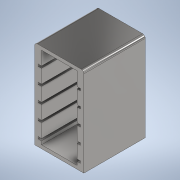
# Autodesk Inventor part: RackV2
Saved by Autodesk Inventor 2021 (Build 250183000, 183)
## iProperties
Created: 2023-04-06
Part Number: RackV2
Material: Steel
Document SubType Name: Modeling
Designer: EF0481
Density: 7.85 g/cm^3
Appearance: Steel - Polished
Author: EF0481
Autodesk Inventor part; units mm, degrees
ref_plane "YZ Plane" through (0, 0, 0) normal (1, 0, 0) x (0, 1, 0)
ref_plane "XZ Plane" through (0, 0, 0) normal (0, 1, 0) x (-1, 0, 0)
ref_plane "XY Plane" through (0, 0, 0) normal (0, 0, 1) x (1, 0, 0)
sketch "Sketch1" plane through (0, 0, 0) normal (0, 0, 1) x (1, 0, 0)
  line L0 (0, 0) -> (72, 0)
  line L1 (72, 0) -> (72, 130)
  line L2 (72, 130) -> (0, 130)
  line L3 (0, 130) -> (0, 0)
  dimension "d0" = 72
  dimension "d1" = 130
  constraints: 8 end point, 2 parallel, 1 horizontal, 1 perpendicular
  measures "d0" distance of L2.end L1.end
  measures "d1" distance of L1.end L0.end
extrude "Extrusion1" add sketch "Sketch1" along normal blind 90
sketch "Sketch2" plane through (0, 0, 90) normal (0, 0, 1) x (1, 0, 0)
  line L0 (10, 125) -> (10, 105)
  line L1 (10, 105) -> (5, 105)
  line L2 (5, 105) -> (5, 102)
  line L3 (5, 102) -> (10, 102)
  line L4 (10, 102) -> (10, 82)
  line L5 (10, 82) -> (5, 82)
  line L6 (5, 82) -> (5, 79)
  line L7 (5, 79) -> (10, 79)
  line L8 (10, 79) -> (10, 59)
  line L9 (10, 59) -> (5, 59)
  line L10 (5, 59) -> (5, 56)
  line L11 (5, 56) -> (10, 56)
  line L12 (10, 56) -> (10, 36)
  line L13 (10, 36) -> (5, 36)
  line L14 (5, 36) -> (5, 33)
  line L15 (5, 33) -> (10, 33)
  line L16 (10, 33) -> (10, 13)
  line L17 (10, 13) -> (5, 13)
  line L18 (5, 13) -> (5, 10)
  line L19 (5, 10) -> (10, 10)
  line L20 (10, 79.6722) -> (10, 76.6722)
  line L21 (10, 125) -> (62, 125) projected
  line L22 (62, 5) -> (10, 5) projected
  line L23 (62, 105) -> (67, 105)
  line L24 (67, 105) -> (67, 102)
  line L25 (67, 102) -> (62, 102)
  line L26 (62, 82) -> (67, 82)
  line L27 (67, 82) -> (67, 79)
  line L28 (67, 79) -> (62, 79)
  line L29 (62, 59) -> (67, 59)
  line L30 (67, 59) -> (67, 56)
  line L31 (67, 56) -> (62, 56)
  line L32 (62, 36) -> (67, 36)
  line L33 (67, 36) -> (67, 33)
  line L34 (67, 33) -> (62, 33)
  line L35 (62, 13) -> (67, 13)
  line L36 (67, 13) -> (67, 10)
  line L37 (67, 10) -> (62, 10)
  line L38 (10, 125) -> (62, 125)
  line L39 (62, 125) -> (62, 105)
  line L40 (62, 102) -> (62, 82)
  line L41 (62, 79) -> (62, 59)
  line L42 (62, 56) -> (62, 36)
  line L43 (62, 33) -> (62, 13)
  line L44 (62, 10) -> (62, 5)
  line L45 (10, 10) -> (10, 5)
  point P0 (0, 0)
  dimension "d7" = 20
  dimension "d8" = 5
  dimension "d9" = 3
  dimension "d10" = 20
  dimension "d11" = 5
  dimension "d12" = 3
  dimension "d13" = 20
  dimension "d14" = 3
  dimension "d15" = 20
  dimension "d16" = 5
  dimension "d17" = 3
  dimension "d18" = 20
  dimension "d19" = 3
  dimension "d20" = 3
  constraints: 88 end point, 8 perpendicular, 6 point on line, 4 collinear, 3 vertical, 1 horizontal
  measures "d7" distance of L0.start L0.end
  measures "d8" distance of L0.end L1.end
  measures "d9" distance of L1.end L2.end
  measures "d10" distance of L3.end L4.end
  measures "d11" distance of L4.end L5.end
  measures "d12" distance of L5.end L6.end
  measures "d13" distance of L7.end L8.end
  measures "d14" distance of L9.end L10.end
  measures "d15" distance of L11.end L12.end
  measures "d16" distance of L12.end L13.end
  measures "d17" distance of L13.end L14.end
  measures "d18" distance of L15.end L16.end
  measures "d19" distance of L17.end L18.end
  measures "d20" distance of L20.start L20.end
extrude "Extrusion2" cut sketch "Sketch2" against normal blind 90
fillet "Fillet1" radius 4 2 edges at (72, 130, 45) (0, 130, 45)
sketch "Sketch3" plane through (0, 0, 0) normal (0, 0, -1) x (-1, 0, 0)
  circle A0 centre (-67, 125) radius 1.5
  line L0 (-72, 126) -> (-72, 0)
  line L1 (-4, 130) -> (-68, 130)
  line L2 (0, 0) -> (0, 126)
  arc A1 (0, 126) -> (-4, 130) centre (-4, 126) ccw
  line L3 (-4, 130) -> (-68, 130)
  arc A2 (-68, 130) -> (-72, 126) centre (-68, 126) ccw
  line L4 (-72, 126) -> (-72, 0)
  line L5 (-72, 0) -> (0, 0)
  line L6 (0, 0) -> (0, 126)
  line L7 (-68, 130) -> (-4, 130)
  line L8 (0, 0) -> (-72, 0)
  circle A3 centre (-5, 125) radius 1.5
  circle A4 centre (-67, 5) radius 1.5
  circle A5 centre (-5, 5) radius 1.5
  dimension "d24" = 3
  dimension "d25" = 5
  dimension "d26" = 5
  dimension "d27" = 3
  dimension "d28" = 5
  dimension "d29" = 5
  constraints: 18 end point, 6 centre point, 4 point on circle
  measures "d24" diameter of A0
  measures "d25" distance from line of L0 A0.centre
  measures "d26" distance from line of L1 A0.centre
  measures "d27" diameter of A4
  measures "d28" distance from line of A4.centre L0
  measures "d29" distance from line of L5 A4.centre
hole "Hole1" at (67, 125, 0) at (5, 125, 0) at (5, 5, 0) at (67, 5, 0) direction (0, 0, 1) diameter 2.6416 depth 10.979 thread size "6-32 UNC" class "2B" standard "ANSI Unified Screw Threads"
sketch "Sketch4" plane through (0, 0, 0) normal (0, 0, -1) x (-1, 0, 0)
  point P0 (0, 0)
body "Solid1"
